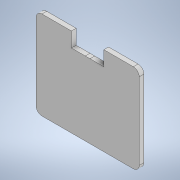
# Autodesk Inventor part: pcb_balun_top
Saved by Autodesk Inventor 2020.2 (Build 242310000, 310)
## iProperties
Created: 2020-09-26
Part Number: pcb_balun_top
Material: Generic
Document SubType Name: Modeling
Designer: Krishna Makhija
Density: 1 g/cm^3
Appearance: Default
Author: Krishna Makhija
Autodesk Inventor part; units mm, degrees
ref_plane "YZ Plane" through (0, 0, 0) normal (1, 0, 0) x (0, 1, 0)
ref_plane "XZ Plane" through (0, 0, 0) normal (0, 1, 0) x (-1, 0, 0)
ref_plane "XY Plane" through (0, 0, 0) normal (0, 0, 1) x (1, 0, 0)
sketch "Sketch1" plane through (0, 0, 0) normal (0, 0, 1) x (1, 0, 0)
  line L0 (17.5001, -12.5) -> (-17.4999, -12.5)
  line L1 (17.5001, -12.5) -> (-17.4999, 12.4999) construction
  line L2 (-17.4999, -12.5) -> (17.5001, 12.5002) construction
  line L3 (-17.4999, 17.4999) -> (-5.4995, 17.4999)
  line L4 (-17.4999, 5.0001) -> (-17.4999, 17.4999)
  line L5 (5.5001, 17.4996) -> (17.5001, 17.4996)
  line L6 (17.5001, 17.4996) -> (17.5001, 5.0001)
  line L7 (-0.7998, 12.4999) -> (-5.4995, 12.5011)
  line L8 (0.7998, 12.4999) -> (5.5001, 12.4999)
  line L9 (-5.4995, 17.4999) -> (-5.4995, 12.5011)
  line L10 (5.5001, 17.4996) -> (5.5001, 12.4999)
  line L11 (-17.4999, -12.5) -> (-17.4999, 5.0001)
  line L12 (17.5001, -12.5) -> (17.5001, 5.0001)
  line L13 (-0.7998, 12.4999) -> (0.7998, 12.4999)
  point P0 (0, 0)
  constraints: 28 end point, 4 horizontal, 2 parallel, 2 point on line, 2 vertical, 1 perpendicular
extrude "Extrusion1" add sketch "Sketch1" along normal blind 1.6
fillet "Fillet2" radius 2 4 edges at (17.5001, 17.4996, 0.8) (17.5001, -12.5, 0.8) (-17.4999, -12.5, 0.8) (-17.4999, 17.4999, 0.8)
body "Solid1"
